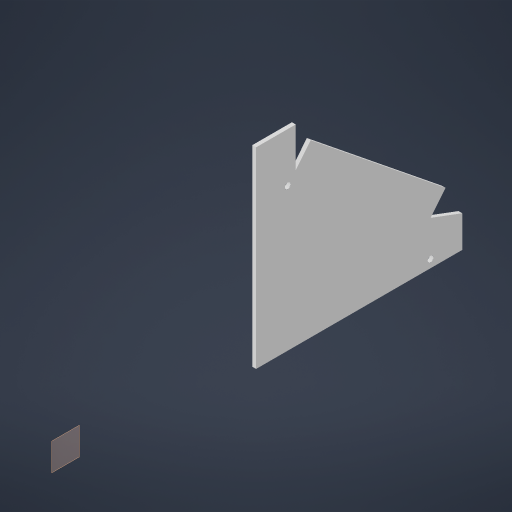
# Autodesk Inventor part: backpanel
Saved by Autodesk Inventor 2024 (Build 280153000, 153)
## iProperties
Created: 2023-11-22
Part Number: backpanel
Material: Generic
Document SubType Name: Sheet Metal
Designer: reima
Density: 1 g/cm^3
Appearance: Default
Sheet Metal Rule: Default
Author: reima
Autodesk Inventor part; units mm, degrees
ref_plane "YZ Plane" through (0, 0, 0) normal (1, 0, 0) x (0, 1, 0)
ref_plane "XZ Plane" through (0, 0, 0) normal (0, 1, 0) x (-1, 0, 0)
ref_plane "XY Plane" through (0, 0, 0) normal (0, 0, 1) x (1, 0, 0)
sketch "Sketch1" plane through (0, 0, 0) normal (1, 0, 0) x (0, 1, 0)
  line L0 (6.0871, 13.8808) -> (-19.3129, 13.8808)
  line L1 (-19.3129, 13.8808) -> (-19.3129, -316.3192)
  line L2 (-19.3129, -316.3192) -> (6.0871, -316.3192)
  line L3 (6.0871, -316.3192) -> (6.0871, 13.8808)
  circle A0 centre (-12.9629, -11.5192) radius 2.3368
  circle A1 centre (-12.9629, -290.9192) radius 2.3368
  line L4 (-19.3129, -151.2192) -> (65.5988, -151.2192) construction
  circle A2 centre (94.9871, -125.8192) radius 2.3368
  circle A3 centre (94.9871, -176.6192) radius 2.3368
  line L5 (94.9871, -125.8192) -> (94.9871, -176.6192) construction
  line L6 (-12.9629, -11.5192) -> (-12.9629, -290.9192) construction
  line L7 (102.6071, -119.4692) -> (102.6071, -182.9692)
  line L8 (6.0871, -11.5192) -> (15.6121, -11.5192) construction
  line L9 (6.0871, -290.9192) -> (15.6121, -290.9192) construction
  line L10 (6.0871, 13.8808) -> (15.6121, -11.5192)
  line L11 (6.0871, -316.3192) -> (15.6121, -290.9192)
  line L12 (102.6071, -119.4692) -> (15.6121, -11.5192)
  line L13 (102.6071, -182.9692) -> (15.6121, -290.9192)
  line L14 (102.6071, -119.4692) -> (134.3571, -119.4692)
  line L15 (134.3571, -119.4692) -> (134.3571, -182.9692)
  line L16 (134.3571, -182.9692) -> (102.6071, -182.9692)
  line L17 (102.6071, -182.9692) -> (102.6071, -119.4692)
  line L18 (102.6071, -182.9692) -> (117.44, -194.9228)
  line L19 (15.6121, -290.9192) -> (30.445, -302.8728)
  line L20 (117.44, -194.9228) -> (30.445, -302.8728)
  line L21 (102.6071, -119.4692) -> (117.44, -107.5156)
  line L22 (117.44, -107.5156) -> (30.445, 0.4344)
  line L23 (30.445, 0.4344) -> (15.6121, -11.5192)
  point P0 (0, 0)
  dimension "d0" = 25.4
  dimension "d1" = 330.2
  dimension "d2" = 4.6736
  dimension "d3" = 4.6736
  dimension "d4" = 279.4
  dimension "d5" = 25.4
  dimension "d6" = 6.35
  dimension "d7" = 84.9117
  dimension "d8" = 4.6736
  dimension "d9" = 4.6736
  dimension "d10" = 50.8
  dimension "d11" = 25.4
  dimension "d12" = 107.95
  dimension "d13" = 7.62
  dimension "d14" = 9.525
  dimension "d15" = 9.525
  dimension "d16" = 63.5
  dimension "d17" = 6.35
  dimension "d18" = 31.75
  dimension "d19" = 19.05
  dimension "d20" = 19.05
  constraints: 48 end point, 7 perpendicular, 4 centre point, 4 horizontal, 4 parallel, 3 vertical, 2 point on line, 1 midpoint
  measures "d0" distance of L2.end L1.end
  measures "d1" distance of L1.end L0.end
  measures "d2" diameter of A0
  measures "d3" diameter of A1
  measures "d4" distance of L6.end L6.start
  measures "d5" distance from line of L2 L6.end
  measures "d6" distance from line of L1 L6.end
  measures "d7" distance of L4.start L4.end
  measures "d8" diameter of A2
  measures "d9" diameter of A3
  measures "d10" distance of L5.end L5.start
  measures "d11" distance from line of L4 L5.start
  measures "d12" distance from line of L6 L5.start
  measures "d13" distance between parallel lines of L5 L7
  measures "d14" distance of L8.start L8.end
  measures "d15" distance of L9.start L9.end
  measures "d16" distance of L7.start L7.end
  measures "d17" vertical distance of L5.end L7.end
  measures "d18" distance of L15.end L16.end
  measures "d19" distance of L16.end L18.end
  measures "d20" distance of L7.start L21.end
ref_plane "Work Plane1" through (1.5875, 0, 0) normal (1, 0, 0) x (0, 0, -1)
extrude "Plate1" add sketch "Sketch1" along normal blind 3.048
sketch "Sketch3" plane through (0, 0, 0) normal (-1, 0, 0) x (0, 0, 1)
  circle A0 centre (-176.6192, 94.9871) radius 2.3368 projected
  circle A1 centre (-125.8192, 94.9871) radius 2.3368 projected
  circle A2 centre (-11.5192, -12.9629) radius 2.3368 projected
  circle A3 centre (-290.9192, -12.9629) radius 2.3368 projected
  line L0 (-107.5156, 117.44) -> (0.4344, 30.445) projected
  line L1 (-119.4692, 102.6071) -> (-107.5156, 117.44) projected
  line L2 (-119.4692, 134.3571) -> (-119.4692, 102.6071) projected
  line L3 (-182.9692, 134.3571) -> (-119.4692, 134.3571) projected
  line L4 (-182.9692, 102.6071) -> (-182.9692, 134.3571) projected
  line L5 (-194.9228, 117.44) -> (-182.9692, 102.6071) projected
  line L6 (-302.8728, 30.445) -> (-194.9228, 117.44) projected
  line L7 (-290.9192, 15.6121) -> (-302.8728, 30.445) projected
  line L8 (-316.3192, 6.0871) -> (-290.9192, 15.6121) projected
  line L9 (-316.3192, -19.3129) -> (-316.3192, 6.0871) projected
  line L10 (13.8808, -19.3129) -> (-316.3192, -19.3129) projected
  line L11 (13.8808, 6.0871) -> (13.8808, -19.3129) projected
  line L12 (-11.5192, 15.6121) -> (13.8808, 6.0871) projected
  line L13 (0.4344, 30.445) -> (-11.5192, 15.6121) projected
  line L14 (-151.2192, 134.3571) -> (-151.2192, -19.3129)
  point P0 (0, 0)
  constraints: 2 end point, 2 midpoint
extrude "Cut1" cut sketch "Sketch3" against normal blind 3.048 contours L0 L13 L12 L11 L10 L14 L3 L2 L1
equation "\"d24\" = Thickness"
equation "\"d23\" = Thickness"
equation "\"BendRadius\" = Thickness"
equation "\"BendReliefWidth\" = Thickness"
equation "\"BendReliefDepth\" = 0.5 * Thickness"
equation "\"CornerReliefSize\" = 4 * Thickness"
equation "\"MinimumRemnant\" = 2 * Thickness"
equation "\"TransitionRadius\" = BendRadius"
equation "\"JacobiRadiusSize\" = BendRadius"
equation "\"GapSize\" = Thickness"
equation "\"Thickness\" = 3.048"
body "Solid2"
